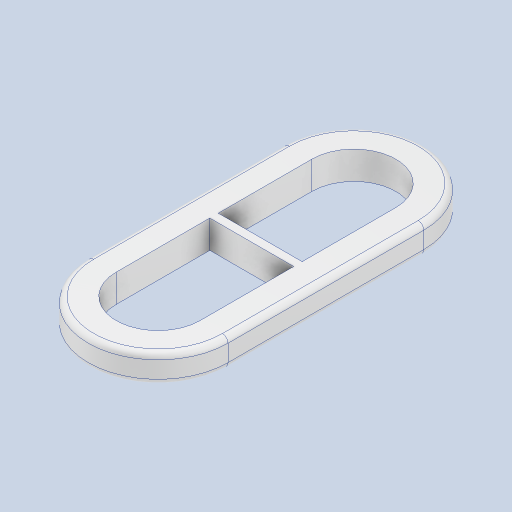
# Autodesk Inventor part: mod2
Saved by Autodesk Inventor 2024 (Build 280153000, 153)
## iProperties
Created: 2025-12-02
Part Number: mod2
Material: Aluminio 6061
Document SubType Name: Modeling
Designer: ANDRES
Density: 2.7 g/cm^3
Appearance: Aluminio - Plano
Author: ANDRES
Autodesk Inventor part; units mm, degrees
ref_plane "YZ Plane" through (0, 0, 0) normal (1, 0, 0) x (0, 1, 0)
ref_plane "XZ Plane" through (0, 0, 0) normal (0, 1, 0) x (-1, 0, 0)
ref_plane "XY Plane" through (0, 0, 0) normal (0, 0, 1) x (1, 0, 0)
sketch "Boceto1" plane through (0, 0, 0) normal (0, 1, 0) x (-1, 0, 0)
  line L0 (0, 35) -> (0, -35) construction
  line L1 (25, 35) -> (25, -35)
  line L2 (-25, -35) -> (-25, 35)
  arc A0 (25, 35) -> (-25, 35) centre (0, 35) ccw
  arc A1 (-25, -35) -> (25, -35) centre (0, -35) ccw
  circle A2 centre (0, -35) radius 15
  circle A3 centre (0, 35) radius 15
  line L3 (0, -20) -> (0, -20)
  line L4 (15, -35) -> (-15, -35)
  line L5 (94.5074, 0) -> (-76.0102, 0) construction
  line L6 (15, 35) -> (-15, 35)
  line L7 (15, -35) -> (-15, -35)
  line L8 (-15, -35) -> (-15, -1.5)
  line L9 (-15, -1.5) -> (15, -1.5)
  line L10 (15, -1.5) -> (15, -35)
  line L11 (-15, 35) -> (-15, 1.5)
  line L12 (-15, 1.5) -> (15, 1.5)
  line L13 (15, 1.5) -> (15, 35)
  point P0 (0, 0)
  point P1 (0, 60)
  point P2 (0, -60)
  point P3 (0, -20)
  point P4 (15, 35)
  point P5 (15, 35)
  dimension "largo" = 120
  dimension "d1" = 50
  dimension "espesor_junta" = 10
  dimension "d3" = 10
  dimension "d6" = 0
  dimension "d9" = 1.5
  constraints: 30 end point, 10 point on circle, 5 symmetric about line, 4 centre point, 4 tangent, 3 horizontal, 3 midpoint, 3 parallel, 2 concentric, 2 vertical, 1 perpendicular, 1 vertical alignment
  measures "largo" distance of point (0, 60) point (0, -60)
  measures "d1" distance between parallel lines of L2 L1
  measures "espesor_junta" radial gap between concentric circles of A1 A2
  measures "d3" radial gap between concentric circles of A0 A3
  measures "d6" distance of L3.start L3.end
  measures "d9" distance between parallel lines of L5 L9
extrude "Extrusión2" add sketch "Boceto1" along normal blind 10
fillet "Empalme1" radius 2 8 edges at (0, 10, 60) (25, 10, 0) (0, 10, -60) (-25, 10, 0) (0, 0, -60) (-25, 0, 0) (0, 0, 60) (25, 0, 0)
equation "\"d3\" = espesor_junta"
